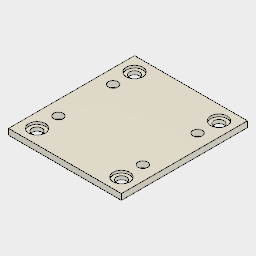
Second Plate v2 (Autodesk Fusion 360 design; units mm, degrees)
Autodesk Fusion 360 part; units mm, degrees
sketch "Sketch1" plane through (0, 0, 0) normal (0, 1, 0) x (1, 0, 0)
  line L0 (0, 0) -> (95, 0)
  line L1 (0, 0) -> (0, 106)
  line L2 (0, 106) -> (95, 106)
  line L3 (95, 106) -> (95, 0)
  line L4 (95, 106) -> (83, 106)
  circle A0 centre (83, 94) radius 7
  line L5 (0, 106) -> (12, 106)
  circle A1 centre (12, 94) radius 7
  circle A2 centre (83, 76) radius 4
  circle A3 centre (12, 76) radius 4
  circle A4 centre (83, 30) radius 4
  circle A5 centre (83, 12) radius 7
  circle A6 centre (12, 30) radius 4
  circle A7 centre (12, 12) radius 7
  circle A8 centre (83, 94) radius 4.25
  circle A9 centre (12, 94) radius 4.25
  circle A10 centre (12, 12) radius 4.25
  circle A11 centre (83, 12) radius 4.25
  dimension "d26" = 8.5
  dimension "d27" = 8.5
  dimension "d28" = 8.5
  measures "d26" diameter of A9
  measures "d27" diameter of A10
  measures "d28" diameter of A11
extrude "Extrude1" add sketch "Sketch1" along normal blind 5 contours L0 L1 L2 L3 L4 L5 | A0 | A1 | A5 | A7
sketch "Sketch2" plane through (0, 5, 0) normal (0, 1, 0) x (-1, 0, 0)
  circle A0 centre (-12, -94) radius 4.25
  circle A1 centre (-83, -76) radius 4
  circle A2 centre (-83, -94) radius 4.25
  circle A3 centre (-12, -76) radius 4
  circle A4 centre (-83, -30) radius 4
  circle A5 centre (-12, -30) radius 4
  circle A6 centre (-83, -12) radius 4.25
  circle A7 centre (-12, -12) radius 4.25
  line L0 (0, 0) -> (-95, 0)
  line L1 (-95, 0) -> (-95, -106)
  line L2 (-95, -106) -> (0, -106)
  line L3 (0, -106) -> (0, 0)
  circle A8 centre (-12, -12) radius 7
  circle A9 centre (-83, -12) radius 7
  circle A10 centre (-83, -94) radius 7
  circle A11 centre (-12, -94) radius 7
  dimension "d31" = 14
  dimension "d32" = 14
  dimension "d33" = 14
  dimension "d34" = 14
  measures "d31" diameter of A8
  measures "d32" diameter of A9
  measures "d33" diameter of A10
  measures "d34" diameter of A11
extrude "Extrude2" cut sketch "Sketch2" against normal blind 2 contours A8 | A9 | A10 | A11
